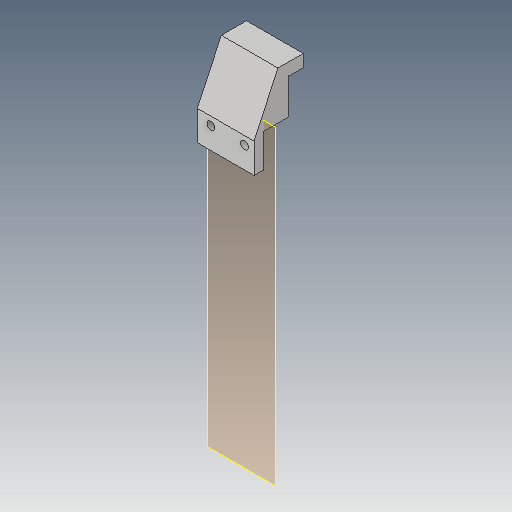
# Autodesk Inventor part: OPENTRONS_Autofocus_NEMA_holder_tmp
Saved by Autodesk Inventor 2019.4 (Build 234330000, 330)
## iProperties
Created: 2021-01-06
Part Number: OPENTRONS_Autofocus_NEMA_holder_tmp
Material: Generic
Document SubType Name: Modeling
Designer: diederichbenedict
Density: 1 g/cm^3
Appearance: Default
Author: diederichbenedict
Autodesk Inventor part; units mm, degrees
ref_plane "YZ Plane" through (0, 0, 0) normal (1, 0, 0) x (0, 1, 0)
ref_plane "XZ Plane" through (0, 0, 0) normal (0, 1, 0) x (-1, 0, 0)
ref_plane "Work Plane1" through (0, 0, 0) normal (0, 0, 1) x (1, 0, 0)
sketch "Sketch1" plane through (0, 0, 0) normal (0, 0, 1) x (1, 0, 0)
  circle A0 centre (11, 82.9899) radius 1.6 projected
  circle A1 centre (-3, 82.9899) radius 1.6 projected
  circle A2 centre (7.5, 24) radius 6.4506 projected
  circle A3 centre (7.5, 64) radius 6.4305 projected
  arc A4 (0, 42.6389) -> (0, 45.3611) centre (-0.5, 44) ccw projected
  line L0 (0, -32) -> (0, 42.6389) projected
  line L1 (0, -32) -> (15, -32) projected
  line L2 (15, 35.9533) -> (15, -32) projected
  arc A5 (15, 35.9533) -> (15, 52.0467) centre (7.5, 44) ccw projected
  line L3 (15, 52.0467) -> (15, 86) projected
  line L4 (0, 45.3611) -> (0, 74) projected
  circle A6 centre (7.5, 36) radius 1.45 projected
  circle A7 centre (7.5, 52) radius 1.45 projected
  circle A8 centre (15.5, 44) radius 1.45 projected
  circle A9 centre (7.5, 44) radius 6 projected
  line L5 (-6.6903, 74) -> (15, 74)
  line L6 (15, 74) -> (15, 107.8848)
  line L7 (15, 107.8848) -> (-6.6903, 107.8848)
  line L8 (-6.6903, 107.8848) -> (-6.6903, 74)
  line L9 (15, 86) -> (-7, 86) projected
  line L10 (-7, 86) -> (-7, 74) projected
  line L11 (-7, 74) -> (0, 74) projected
  point P0 (0, 0)
  constraints: 8 end point, 2 parallel, 1 horizontal, 1 perpendicular
extrude "Extrusion1" add sketch "Sketch1" along normal blind 4 contours L5 L8 L9 L3 | L8 L7 L6 L9
sketch "Sketch2" plane through (0, 0, 0) normal (0, 0, -1) x (-1, 0, 0)
  circle A0 centre (3, 82.9899) radius 1.6 projected
  circle A1 centre (-11, 82.9899) radius 1.6 projected
  line L0 (6.6903, 74) -> (6.6903, 107.8848) projected
  line L1 (6.6903, 107.8848) -> (-15, 107.8848) projected
  line L2 (-15, 107.8848) -> (-15, 74) projected
  line L3 (-15, 74) -> (6.6903, 74) projected
  line L4 (-15, 74) -> (-15, 107.8848) projected
  line L5 (-15, 107.8848) -> (6.6903, 107.8848)
  line L6 (6.6903, 107.8848) -> (6.6903, 87.9676)
  line L7 (6.6903, 87.9676) -> (-15, 87.9676)
  line L8 (-15, 87.9676) -> (-15, 107.8848)
  point P0 (0, 0)
  constraints: 8 end point, 2 parallel, 1 horizontal, 1 perpendicular, 1 point on line
ref_plane "Work Plane2" through (-7, 76.75, -10.5439) normal (0, 0, 1) x (1, 0, 0)
extrude "Extrusion2" add sketch "Sketch2" along normal up to surface (10.5439 mm away) contours L7 L2 L1 L0
sketch "Sketch3" plane through (15, 87.9676, -10.5439) normal (0, 0, -1) x (-1, 0, 0)
  line L0 (0, 19.9172) -> (0, 0) projected
  line L1 (0, 0) -> (21.6903, 0) projected
  line L2 (21.6903, 0) -> (21.6903, 19.9172) projected
  line L3 (21.6903, 19.9172) -> (0, 19.9172) projected
  line L4 (0, 19.9172) -> (21.6903, 19.9172) projected
  line L5 (0, -13.9676) -> (0, 19.9172) projected
  line L6 (21.6903, 19.9172) -> (0, 19.9172)
  line L7 (0, 19.9172) -> (0, 14.7562)
  line L8 (0, 14.7562) -> (21.6903, 14.7562)
  line L9 (21.6903, 14.7562) -> (21.6903, 19.9172)
  line L10 (21.6903, 0) -> (21.6903, 19.9172) projected
  line L11 (0, 19.9172) -> (0, 0) projected
  line L12 (21.6903, 19.9172) -> (0, 19.9172)
  line L13 (0, 19.9172) -> (0, 14.63)
  line L14 (0, 14.63) -> (21.6903, 14.63)
  line L15 (21.6903, 14.63) -> (21.6903, 19.9172)
  line L16 (22, 14.2824) -> (14.4, 14.2824) projected
  point P0 (15, -87.9676)
  constraints: 16 end point, 4 parallel, 2 horizontal, 2 perpendicular, 2 point on line
extrude "Extrusion3" add sketch "Sketch3" along normal blind 6 contours L3 L2 L8 L0
sketch "Sketch4" plane through (-6.6903, 74, 4) normal (-1, 0, 0) x (0, 0, 1)
  circle A0 centre (-28.5439, 14.25) radius 10.8 projected
  line L0 (-20.5439, 33.8848) -> (-20.5439, 28.7239) projected
  line L1 (0, 0) -> (-20.5439, 0)
  line L2 (-20.5439, 0) -> (-20.5439, 33.8848)
  line L3 (-20.5439, 33.8848) -> (0, 33.8848)
  line L4 (0, 33.8848) -> (0, 0)
  circle A1 centre (-17.0439, 25.75) radius 1.1 projected
  line L5 (-14.5439, 25.75) -> (-14.5439, 2.75) projected
  arc A2 (-14.5439, 25.75) -> (-17.0439, 28.25) centre (-17.0439, 25.75) ccw projected
  line L6 (-40.0439, 28.25) -> (-17.0439, 28.25) projected
  arc A3 (-40.0439, 28.25) -> (-42.5439, 25.75) centre (-40.0439, 25.75) ccw projected
  line L7 (-42.5439, 2.75) -> (-42.5439, 25.75) projected
  arc A4 (-42.5439, 2.75) -> (-40.0439, 0.25) centre (-40.0439, 2.75) ccw projected
  line L8 (-17.0439, 0.25) -> (-40.0439, 0.25) projected
  arc A5 (-17.0439, 0.25) -> (-14.5439, 2.75) centre (-17.0439, 2.75) ccw projected
  circle A6 centre (-28.5439, 14.25) radius 11 projected
  circle A7 centre (-40.0439, 25.75) radius 1.025 projected
  circle A8 centre (-17.0439, 25.75) radius 1.025 projected
  circle A9 centre (-17.0439, 2.75) radius 1.025 projected
  circle A10 centre (-40.0439, 2.75) radius 1.025 projected
  line L9 (0, 33.8848) -> (0, 0) projected
  point P0 (-4, -74)
  constraints: 8 end point, 2 parallel, 1 horizontal, 1 perpendicular
extrude "Extrusion4" add sketch "Sketch4" along normal blind 2 contours A0 L2 | A0 L2 A6 | L2 L6 A2 L5 A5 L8 A6 | L2 L0 L3 L4 L1 L8 A5 L5 A2 L6 picked at (-19.7185, 15.1251) picked at (-18.4698, 18.1768)
sketch "Sketch5" plane through (-8.6903, 74, 4) normal (-1, 0, 0) x (0, 0, 1)
  circle A0 centre (-28.5439, 14.25) radius 11 projected
  circle A1 centre (-28.5439, 14.25) radius 11.9547
  point P0 (-4, -74)
  constraints: 1 centre point, 1 coincident
extrude "Extrusion5" cut sketch "Sketch5" against normal blind 2 contours A0 | A1
chamfer "Chamfer1" distance 10 angle 65 1 edges at (3.1548, 107.8848, 4) measured on face at (7.1032, 107.8848, -2.848)
body "Solid1"
